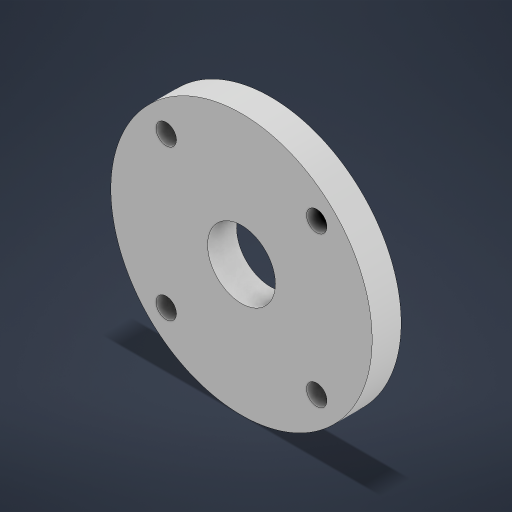
# Autodesk Inventor part: Stage2MotorSpacer
Saved by Autodesk Inventor 2024 (Build 280153000, 153)
## iProperties
Created: 2024-02-26
Part Number: Stage2MotorSpacer
Material: Generic
Document SubType Name: Modeling
Designer: avsar
Density: 1 g/cm^3
Appearance: Default
Author: avsar
Autodesk Inventor part; units mm, degrees
ref_plane "YZ Plane" through (0, 0, 0) normal (1, 0, 0) x (0, 1, 0)
ref_plane "XZ Plane" through (0, 0, 0) normal (0, 1, 0) x (-1, 0, 0)
ref_plane "XY Plane" through (0, 0, 0) normal (0, 0, 1) x (1, 0, 0)
sketch "Sketch1" plane through (0, 0, 0) normal (0, 0, 1) x (1, 0, 0)
  circle A0 centre (0, 0) radius 27
  circle A1 centre (-15.5563, 15.5563) radius 2.1
  line L0 (-15.5563, 15.5563) -> (0, 0) construction
  line L1 (0, 0) -> (-27, 0) construction
  circle A2 centre (-15.5563, -15.5563) radius 2.1
  circle A3 centre (15.5563, -15.5563) radius 2.1
  circle A4 centre (15.5563, 15.5563) radius 2.1
  dimension "d0" = 54
  dimension "d1" = 4.2
  dimension "d2" = 22
  dimension "d3" = 45
  dimension "d6" = 360
  constraints: 4 centre point, 4 end point, 1 coincident, 1 horizontal, 1 horizontal alignment, 11 other
  measures "d1" diameter of A1
  measures "d2" distance of L0.start L0.end
  measures "d3" angle of L1 L0
extrude "Extrusion1" add sketch "Sketch1" along normal blind 6
sketch "Sketch2" plane through (0, 0, 6) normal (0, 0, 1) x (1, 0, 0)
  circle A0 centre (0, 0) radius 7
  dimension "d10" = 14
  constraints: 1 centre point, 1 coincident
  measures "d10" diameter of A0
extrude "Extrusion2" cut sketch "Sketch2" against normal through all
body "Solid1"
